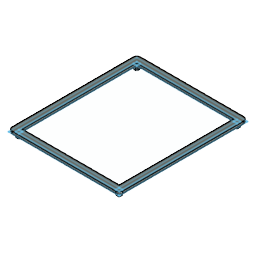
radpad_top (Autodesk Fusion 360 design; units mm, degrees)
part number: 2026-05-31-13-12-00-221
Autodesk Fusion 360 part; units mm, degrees
sketch "Sketch1" plane through (0, 0, 0) normal (0, 0, 1) x (1, 0, 0)
  line L0 (-77.6757, 64.539) -> (16.5243, 64.539)
  line L1 (16.5243, 64.539) -> (16.5243, -44.661)
  line L2 (16.5243, -44.661) -> (-77.6757, -44.661)
  line L3 (-77.6757, -44.661) -> (-77.6757, 64.539)
  line L4 (-74.6757, 61.539) -> (13.5243, 61.539)
  line L5 (13.5243, 61.539) -> (13.5243, -41.661)
  line L6 (13.5243, -41.661) -> (-74.6757, -41.661)
  line L7 (-74.6757, -41.661) -> (-74.6757, 61.539)
  line L8 (-74.6757, 61.539) -> (-71.8757, 61.539)
  line L9 (-71.8757, 61.539) -> (-71.8757, 58.739)
  line L10 (-71.8757, 58.739) -> (-74.6757, 58.739)
  line L11 (-74.6757, 58.739) -> (-74.6757, 61.539)
  line L12 (13.5243, 61.539) -> (10.7243, 61.539)
  line L13 (10.7243, 61.539) -> (10.7243, 58.739)
  line L14 (10.7243, 58.739) -> (13.5243, 58.739)
  line L15 (13.5243, 58.739) -> (13.5243, 61.539)
  line L16 (-74.6757, -41.661) -> (-71.8757, -41.661)
  line L17 (-71.8757, -41.661) -> (-71.8757, -38.861)
  line L18 (-71.8757, -38.861) -> (-74.6757, -38.861)
  line L19 (-74.6757, -38.861) -> (-74.6757, -41.661)
  line L20 (13.5243, -41.661) -> (10.7243, -41.661)
  line L21 (10.7243, -41.661) -> (10.7243, -38.861)
  line L22 (10.7243, -38.861) -> (13.5243, -38.861)
  line L23 (13.5243, -38.861) -> (13.5243, -41.661)
  line L24 (-71.8757, -38.861) -> (10.7243, -38.861)
  line L25 (10.7243, -38.861) -> (10.7243, -41.661)
  line L26 (10.7243, -41.661) -> (-71.8757, -41.661)
  line L27 (-71.8757, -41.661) -> (-71.8757, -38.861)
  line L28 (-71.8757, 58.739) -> (10.7243, 58.739)
  line L29 (10.7243, 58.739) -> (10.7243, 61.539)
  line L30 (10.7243, 61.539) -> (-71.8757, 61.539)
  line L31 (-71.8757, 61.539) -> (-71.8757, 58.739)
  line L32 (-71.8757, 58.739) -> (-74.6757, 58.739)
  line L33 (-74.6757, 58.739) -> (-74.6757, -38.861)
  line L34 (-74.6757, -38.861) -> (-71.8757, -38.861)
  line L35 (-71.8757, -38.861) -> (-71.8757, 58.739)
  line L36 (13.5243, -38.861) -> (10.7243, -38.861)
  line L37 (10.7243, -38.861) -> (10.7243, 58.739)
  line L38 (10.7243, 58.739) -> (13.5243, 58.739)
  line L39 (13.5243, 58.739) -> (13.5243, -38.861)
  dimension "d1" = 94.2
  dimension "d2" = 109.2
  dimension "d3" = 88.2
  dimension "d4" = 103.2
  dimension "d5" = 3
  dimension "d6" = 3
  dimension "d7" = 2.8
  dimension "d8" = 2.8
  dimension "d9" = 2.8
  dimension "d10" = 2.8
  dimension "d11" = 2.8
  dimension "d12" = 2.8
  dimension "d13" = 2.8
  dimension "d14" = 2.8
  constraint horizontal L0
  constraint vertical L1
  constraint horizontal L2
  constraint vertical L3
  constraint horizontal L4
  constraint vertical L5
  constraint horizontal L6
  constraint vertical L7
  constraint horizontal L8
  constraint vertical L9
  constraint horizontal L10
  constraint vertical L11
  constraint horizontal L12
  constraint vertical L13
  constraint horizontal L14
  constraint vertical L15
  constraint horizontal L16
  constraint vertical L17
  constraint horizontal L18
  constraint vertical L19
  constraint horizontal L20
  constraint vertical L21
  constraint horizontal L22
  constraint vertical L23
  constraint horizontal L24
  constraint vertical L25
  constraint horizontal L26
  constraint vertical L27
  constraint horizontal L28
  constraint vertical L29
  constraint horizontal L30
  constraint vertical L31
  constraint horizontal L32
  constraint vertical L33
  constraint horizontal L34
  constraint vertical L35
  constraint horizontal L36
  constraint vertical L37
  constraint horizontal L38
  constraint vertical L39
  measures "d1" distance of L0.start L0.end
  measures "d2" distance of L0.start L2.end
  measures "d3" distance of L4.start L4.end
  measures "d4" distance of L4.start L6.end
  measures "d5" distance of L0 L4
  measures "d6" distance of L3 L7
  measures "d7" distance of L4.start L8.end
  measures "d8" distance of L4.start L10.end
  measures "d9" distance of L4.end L12.end
  measures "d10" distance of L4.end L14.end
  measures "d11" distance of L6.end L16.end
  measures "d12" distance of L6.end L18.end
  measures "d13" distance of L5.end L20.end
  measures "d14" distance of L5.end L22.end
extrude "Extrude1" add sketch "Sketch1" along normal blind 2 contours L0 L1 L2 L3 | L4 L7 L8 L9 L10 L11 L31 L32 | L4 L9 L13 L28 L29 L30 L31 | L7 L10 L18 L32 L33 L34 L35 | L4 L5 L12 L13 L14 L15 L29 L38 | L6 L7 L16 L17 L18 L19 L27 L34 | L5 L14 L22 L36 L37 L38 L39 | L6 L17 L21 L24 L25 L26 L27 | L5 L6 L20 L21 L22 L23 L25 L36 makes body 1
extrude "Extrude2" add sketch "Sketch1" against normal blind 4 separate body contours L4 L7 L8 L9 L10 L11 L31 L32 | L4 L5 L12 L13 L14 L15 L29 L38 | L6 L7 L16 L17 L18 L19 L27 L34 | L5 L6 L20 L21 L22 L23 L25 L36 makes body 2 at (13.5243, 60.6057, -1.3333) makes body 3 at (-72.809, -38.861, -1.3333) makes body 4 at (-73.7424, 61.539, -1.3333) makes body 5 at (13.5243, -39.7943, -1.3333)
fillet "Fillet1" radius 3 4 edges at (16.5243, 64.539, 1) (-77.6757, 64.539, 1) (-77.6757, -44.661, 1) (16.5243, -44.661, 1) on bodies 1
fillet "Fillet2" radius 1 4 edges at (10.7243, 58.739, -2) (-71.8757, -38.861, -2) (-71.8757, 58.739, -2) (10.7243, -38.861, -2) on bodies 2 3 4 5
